Autodesk Inventor part; units mm, degrees
(part 4 of 4)
sketch "Эскиз11" plane through (0, 0, 5) normal (0, 0, 1) x (1, 0, 0)
  arc A0 (11.5664, -69.6508) -> (10.9056, -66.9499) centre (8.6538, -68.9321) ccw projected
  line L0 (10.9056, -66.9499) -> (4.435, -59.5991) projected
  arc A1 (-1.9751, -43.3567) -> (4.435, -59.5991) centre (23.7634, -42.5851) ccw projected
  arc A2 (-1.9751, -43.3567) -> (-21.6517, -33.9507) centre (-14.2373, -43.7243) ccw projected
  line L1 (-21.6517, -33.9507) -> (-22.2304, -34.418) projected
  line L2 (-22.2304, -34.418) -> (-22.7798, -34.9196) projected
  line L3 (-22.7798, -34.9196) -> (-23.0908, -35.1013) projected
  line L4 (-23.0908, -35.1013) -> (-23.2505, -35.1358) projected
  line L5 (-23.2505, -35.1358) -> (-23.3841, -35.1446) projected
  line L6 (-23.3841, -35.1446) -> (-23.5038, -35.1394) projected
  line L7 (-23.5038, -35.1394) -> (-23.6142, -35.1248) projected
  line L8 (-23.6142, -35.1248) -> (-23.8163, -35.0762) projected
  line L9 (-23.8163, -35.0762) -> (-24.0007, -35.009) projected
  line L10 (-24.0007, -35.009) -> (-24.1723, -34.9279) projected
  line L11 (-24.1723, -34.9279) -> (-24.3338, -34.8356) projected
  line L12 (-24.3338, -34.8356) -> (-24.6327, -34.6238) projected
  line L13 (-24.6327, -34.6238) -> (-24.9117, -34.3895) projected
  line L14 (-24.9117, -34.3895) -> (-25.2322, -34.2029) projected
  line L15 (-25.2322, -34.2029) -> (-25.5801, -34.0488) projected
  line L16 (-25.5801, -34.0488) -> (-25.9481, -33.9199) projected
  line L17 (-25.9481, -33.9199) -> (-26.3331, -33.8136) projected
  line L18 (-26.3331, -33.8136) -> (-26.733, -33.7285) projected
  line L19 (-26.733, -33.7285) -> (-27.1462, -33.664) projected
  line L20 (-27.1462, -33.664) -> (-27.5715, -33.6196) projected
  line L21 (-27.5715, -33.6196) -> (-28.0079, -33.5952) projected
  line L22 (-28.0079, -33.5952) -> (-28.4544, -33.5907) projected
  line L23 (-28.4544, -33.5907) -> (-28.7953, -33.6003) projected
  line L24 (-28.7953, -33.6003) -> (-29.9133, -35.4362) projected
  line L25 (-29.9133, -35.4362) -> (-29.7654, -35.7435) projected
  line L26 (-29.7654, -35.7435) -> (-29.5565, -36.138) projected
  line L27 (-29.5565, -36.138) -> (-29.3345, -36.5146) projected
  line L28 (-29.3345, -36.5146) -> (-29.0999, -36.8721) projected
  line L29 (-29.0999, -36.8721) -> (-28.8529, -37.2096) projected
  line L30 (-28.8529, -37.2096) -> (-28.5939, -37.5259) projected
  line L31 (-28.5939, -37.5259) -> (-28.3227, -37.8191) projected
  line L32 (-28.3227, -37.8191) -> (-28.0393, -38.087) projected
  line L33 (-28.0393, -38.087) -> (-27.7427, -38.3253) projected
  line L34 (-27.7427, -38.3253) -> (-27.4298, -38.5244) projected
  line L35 (-27.4298, -38.5244) -> (-27.0936, -38.6648) projected
  line L36 (-27.0936, -38.6648) -> (-26.7683, -38.8331) projected
  line L37 (-26.7683, -38.8331) -> (-26.6121, -38.9343) projected
  line L38 (-26.6121, -38.9343) -> (-26.4613, -39.0495) projected
  line L39 (-26.4613, -39.0495) -> (-26.317, -39.1826) projected
  line L40 (-26.317, -39.1826) -> (-26.1811, -39.3398) projected
  line L41 (-26.1811, -39.3398) -> (-26.1175, -39.4312) projected
  line L42 (-26.1175, -39.4312) -> (-26.0579, -39.5351) projected
  line L43 (-26.0579, -39.5351) -> (-26.0044, -39.6579) projected
  line L44 (-26.0044, -39.6579) -> (-25.9617, -39.8156) projected
  line L45 (-25.9617, -39.8156) -> (-25.9805, -40.1753) projected
  line L46 (-25.9805, -40.1753) -> (-26.174, -40.8936) projected
  line L47 (-26.174, -40.8936) -> (-26.3236, -41.6223) projected
  line L48 (-26.3236, -41.6223) -> (-26.4684, -41.9521) projected
  line L49 (-26.4684, -41.9521) -> (-26.5773, -42.0739) projected
  line L50 (-26.5773, -42.0739) -> (-26.6803, -42.1595) projected
  line L51 (-26.6803, -42.1595) -> (-26.7801, -42.2256) projected
  line L52 (-26.7801, -42.2256) -> (-26.878, -42.2788) projected
  line L53 (-26.878, -42.2788) -> (-27.0701, -42.3582) projected
  line L54 (-27.0701, -42.3582) -> (-27.2588, -42.4123) projected
  line L55 (-27.2588, -42.4123) -> (-27.4453, -42.4475) projected
  line L56 (-27.4453, -42.4475) -> (-27.6302, -42.4678) projected
  line L57 (-27.6302, -42.4678) -> (-27.9965, -42.4721) projected
  line L58 (-27.9965, -42.4721) -> (-28.3599, -42.4466) projected
  line L59 (-28.3599, -42.4466) -> (-28.7289, -42.484) projected
  line L60 (-28.7289, -42.484) -> (-29.101, -42.5638) projected
  line L61 (-29.101, -42.5638) -> (-29.4745, -42.6758) projected
  line L62 (-29.4745, -42.6758) -> (-29.8484, -42.8161) projected
  line L63 (-29.8484, -42.8161) -> (-30.2219, -42.9823) projected
  line L64 (-30.2219, -42.9823) -> (-30.5941, -43.173) projected
  line L65 (-30.5941, -43.173) -> (-30.9643, -43.3871) projected
  line L66 (-30.9643, -43.3871) -> (-31.3317, -43.6239) projected
  line L67 (-31.3317, -43.6239) -> (-31.6956, -43.8826) projected
  line L68 (-31.6956, -43.8826) -> (-31.9658, -44.0908) projected
  line L69 (-31.9658, -44.0908) -> (-31.7912, -46.2332) projected
  line L70 (-31.7912, -46.2332) -> (-31.4909, -46.3949) projected
  line L71 (-31.4909, -46.3949) -> (-31.0899, -46.5913) projected
  line L72 (-31.0899, -46.5913) -> (-30.689, -46.7654) projected
  line L73 (-30.689, -46.7654) -> (-30.289, -46.9168) projected
  line L74 (-30.289, -46.9168) -> (-29.8909, -47.0447) projected
  line L75 (-29.8909, -47.0447) -> (-29.4954, -47.1483) projected
  line L76 (-29.4954, -47.1483) -> (-29.1037, -47.2261) projected
  line L77 (-29.1037, -47.2261) -> (-28.7169, -47.2762) projected
  line L78 (-28.7169, -47.2762) -> (-28.3369, -47.2947) projected
  line L79 (-28.3369, -47.2947) -> (-27.9667, -47.2719) projected
  line L80 (-27.9667, -47.2719) -> (-27.6122, -47.1878) projected
  line L81 (-27.6122, -47.1878) -> (-27.2501, -47.1328) projected
  line L82 (-27.2501, -47.1328) -> (-27.0643, -47.1228) projected
  line L83 (-27.0643, -47.1228) -> (-26.8745, -47.1274) projected
  line L84 (-26.8745, -47.1274) -> (-26.6796, -47.1502) projected
  line L85 (-26.6796, -47.1502) -> (-26.4772, -47.1975) projected
  line L86 (-26.4772, -47.1975) -> (-26.372, -47.2341) projected
  line L87 (-26.372, -47.2341) -> (-26.2627, -47.2832) projected
  line L88 (-26.2627, -47.2832) -> (-26.1473, -47.351) projected
  line L89 (-26.1473, -47.351) -> (-26.0201, -47.4535) projected
  line L90 (-26.0201, -47.4535) -> (-25.8238, -47.7556) projected
  line L91 (-25.8238, -47.7556) -> (-25.5582, -48.4504) projected
  line L92 (-25.5582, -48.4504) -> (-25.2509, -49.1279) projected
  line L93 (-25.2509, -49.1279) -> (-25.1742, -49.4799) projected
  line L94 (-25.1742, -49.4799) -> (-25.1907, -49.6424) projected
  line L95 (-25.1907, -49.6424) -> (-25.2237, -49.7722) projected
  line L96 (-25.2237, -49.7722) -> (-25.2656, -49.8844) projected
  line L97 (-25.2656, -49.8844) -> (-25.3136, -49.9849) projected
  line L98 (-25.3136, -49.9849) -> (-25.4222, -50.1621) projected
  line L99 (-25.4222, -50.1621) -> (-25.5431, -50.3167) projected
  line L100 (-25.5431, -50.3167) -> (-25.6733, -50.4549) projected
  line L101 (-25.6733, -50.4549) -> (-25.811, -50.58) projected
  line L102 (-25.811, -50.58) -> (-26.1047, -50.7987) projected
  line L103 (-26.1047, -50.7987) -> (-26.4138, -50.9917) projected
  line L104 (-26.4138, -50.9917) -> (-26.6903, -51.2389) projected
  line L105 (-26.6903, -51.2389) -> (-26.9445, -51.5221) projected
  line L106 (-26.9445, -51.5221) -> (-27.1808, -51.8323) projected
  line L107 (-27.1808, -51.8323) -> (-27.4008, -52.1655) projected
  line L108 (-27.4008, -52.1655) -> (-27.6053, -52.5195) projected
  line L109 (-27.6053, -52.5195) -> (-27.7943, -52.8926) projected
  line L110 (-27.7943, -52.8926) -> (-27.968, -53.2834) projected
  line L111 (-27.968, -53.2834) -> (-28.126, -53.6909) projected
  line L112 (-28.126, -53.6909) -> (-28.2683, -54.1141) projected
  line L113 (-28.2683, -54.1141) -> (-28.3645, -54.4413) projected
  line L114 (-28.3645, -54.4413) -> (-26.964, -56.072) projected
  line L115 (-26.964, -56.072) -> (-26.626, -56.0262) projected
  line L116 (-26.626, -56.0262) -> (-26.1862, -55.9495) projected
  line L117 (-26.1862, -55.9495) -> (-25.7595, -55.8547) projected
  line L118 (-25.7595, -55.8547) -> (-25.347, -55.7421) projected
  line L119 (-25.347, -55.7421) -> (-24.9496, -55.6115) projected
  line L120 (-24.9496, -55.6115) -> (-24.5688, -55.4628) projected
  line L121 (-24.5688, -55.4628) -> (-24.2061, -55.2956) projected
  line L122 (-24.2061, -55.2956) -> (-23.8638, -55.1088) projected
  line L123 (-23.8638, -55.1088) -> (-23.5455, -54.9003) projected
  line L124 (-23.5455, -54.9003) -> (-23.2594, -54.6643) projected
  line L125 (-23.2594, -54.6643) -> (-23.022, -54.3879) projected
  line L126 (-23.022, -54.3879) -> (-22.7614, -54.1305) projected
  line L127 (-22.7614, -54.1305) -> (-22.617, -54.0133) projected
  line L128 (-22.617, -54.0133) -> (-22.4608, -53.9055) projected
  line L129 (-22.4608, -53.9055) -> (-22.2896, -53.8093) projected
  line L130 (-22.2896, -53.8093) -> (-22.0981, -53.7286) projected
  line L131 (-22.0981, -53.7286) -> (-21.9915, -53.6964) projected
  line L132 (-21.9915, -53.6964) -> (-21.8742, -53.6719) projected
  line L133 (-21.8742, -53.6719) -> (-21.741, -53.6589) projected
  line L134 (-21.741, -53.6589) -> (-21.5778, -53.6671) projected
  line L135 (-21.5778, -53.6671) -> (-21.2415, -53.7961) projected
  line L136 (-21.2415, -53.7961) -> (-20.6181, -54.2021) projected
  line L137 (-20.6181, -54.2021) -> (-19.9714, -54.5696) projected
  line L138 (-19.9714, -54.5696) -> (-19.7024, -54.8092) projected
  line L139 (-19.7024, -54.8092) -> (-19.6203, -54.9504) projected
  line L140 (-19.6203, -54.9504) -> (-19.5706, -55.0748) projected
  line L141 (-19.5706, -55.0748) -> (-19.5386, -55.1902) projected
  line L142 (-19.5386, -55.1902) -> (-19.5183, -55.2997) projected
  line L143 (-19.5183, -55.2997) -> (-19.5021, -55.5069) projected
  line L144 (-19.5021, -55.5069) -> (-19.509, -55.7031) projected
  line L145 (-19.509, -55.7031) -> (-19.5331, -55.8914) projected
  line L146 (-19.5331, -55.8914) -> (-19.571, -56.0735) projected
  line L147 (-19.571, -56.0735) -> (-19.68, -56.4231) projected
  line L148 (-19.68, -56.4231) -> (-19.8167, -56.7609) projected
  line L149 (-19.8167, -56.7609) -> (-19.8951, -57.1234) projected
  line L150 (-19.8951, -57.1234) -> (-19.9342, -57.5019) projected
  line L151 (-19.9342, -57.5019) -> (-19.9431, -57.8918) projected
  line L152 (-19.9431, -57.8918) -> (-19.9252, -58.2907) projected
  line L153 (-19.9252, -58.2907) -> (-19.8825, -58.6973) projected
  line L154 (-19.8825, -58.6973) -> (-19.8162, -59.1102) projected
  line L155 (-19.8162, -59.1102) -> (-19.7269, -59.5285) projected
  line L156 (-19.7269, -59.5285) -> (-19.6153, -59.9511) projected
  line L157 (-19.6153, -59.9511) -> (-19.4817, -60.3771) projected
  line L158 (-19.4817, -60.3771) -> (-19.3672, -60.6983) projected
  line L159 (-19.3672, -60.6983) -> (-17.2757, -61.1943) projected
  line L160 (-17.2757, -61.1943) -> (-17.0291, -60.9587) projected
  line L161 (-17.0291, -60.9587) -> (-16.7184, -60.6381) projected
  line L162 (-16.7184, -60.6381) -> (-16.4289, -60.3106) projected
  line L163 (-16.4289, -60.3106) -> (-16.1614, -59.977) projected
  line L164 (-16.1614, -59.977) -> (-15.9167, -59.6378) projected
  line L165 (-15.9167, -59.6378) -> (-15.696, -59.2937) projected
  line L166 (-15.696, -59.2937) -> (-15.5009, -58.9452) projected
  line L167 (-15.5009, -58.9452) -> (-15.3337, -58.5929) projected
  line L168 (-15.3337, -58.5929) -> (-15.1987, -58.2372) projected
  line L169 (-15.1987, -58.2372) -> (-15.106, -57.878) projected
  line L170 (-15.106, -57.878) -> (-15.0764, -57.5149) projected
  line L171 (-15.0764, -57.5149) -> (-15.0169, -57.1535) projected
  line L172 (-15.0169, -57.1535) -> (-14.9689, -56.9737) projected
  line L173 (-14.9689, -56.9737) -> (-14.9059, -56.7947) projected
  line L174 (-14.9059, -56.7947) -> (-14.824, -56.6163) projected
  line L175 (-14.824, -56.6163) -> (-14.7164, -56.4385) projected
  line L176 (-14.7164, -56.4385) -> (-14.6491, -56.3497) projected
  line L177 (-14.6491, -56.3497) -> (-14.5687, -56.261) projected
  line L178 (-14.5687, -56.261) -> (-14.4685, -56.1721) projected
  line L179 (-14.4685, -56.1721) -> (-14.3317, -56.0828) projected
  line L180 (-14.3317, -56.0828) -> (-13.9838, -55.9895) projected
  line L181 (-13.9838, -55.9895) -> (-13.2409, -55.9516) projected
  line L182 (-13.2409, -55.9516) -> (-12.5016, -55.8687) projected
  arc A3 (4.4993, -64.4993) -> (-12.5016, -55.8687) centre (-14.8291, -81.5133) ccw projected
  line L183 (4.4993, -64.4993) -> (7.5502, -67.9652) projected
  arc A4 (8.211, -70.6661) -> (7.5502, -67.9652) centre (5.2984, -69.9474) ccw projected
  line L184 (8.211, -70.6661) -> (3.0154, -91.7239) projected
  line L185 (3.0154, -91.7239) -> (6.1993, -91.4035) projected
  line L186 (6.1993, -91.4035) -> (11.5664, -69.6508) projected
  circle A5 centre (-14.2373, -43.7243) radius 2.5 projected
  circle A6 centre (-8.2184, -38.4544) radius 1.6 projected
  circle A7 centre (-19.5073, -37.7054) radius 1.6 projected
  circle A8 centre (-20.2562, -48.9943) radius 1.6 projected
  circle A9 centre (-8.9673, -49.7433) radius 1.6 projected
  circle A10 centre (-39.9568, -59.168) radius 2.5 projected
  line L187 (-14.2373, -43.7243) -> (-39.9568, -59.168)
  line L188 (-27.0971, -51.4462) -> (-13.5779, -73.9607)
  arc A11 (-31.273, -92.2767) -> (-29.1996, -94.1293) centre (-28.4651, -91.2206) ccw
  line L189 (-31.273, -92.2767) -> (-34.7203, -83.1105)
  arc A12 (-34.7203, -83.1105) -> (-46.0444, -69.8188) centre (-58.8222, -92.1748) ccw
  arc A13 (-30.0531, -66.4077) -> (-30.4253, -85.4702) centre (-6.3234, -76.4059) ccw
  line L190 (-30.4253, -85.4702) -> (-28.7999, -89.7922)
  arc A14 (-28.7999, -89.7922) -> (-26.7265, -91.6448) centre (-25.9919, -88.7361) ccw
  line L191 (-26.7265, -91.6448) -> (-5.6974, -96.9556)
  line L192 (-5.6974, -96.9556) -> (-7.4766, -99.6154)
  line L193 (-7.4766, -99.6154) -> (-29.1996, -94.1293)
  circle A15 centre (-47.4326, -62.0164) radius 1.6 projected
  circle A16 centre (-37.1084, -66.6437) radius 1.6 projected
  circle A17 centre (-32.4811, -56.3196) radius 1.6 projected
  circle A18 centre (-39.9568, -59.168) radius 2.5 projected
  circle A19 centre (-42.8052, -51.6922) radius 1.6 projected
  arc A20 (-41.4259, -46.9885) -> (-28.2942, -62.9735) centre (-39.9568, -59.168) ccw projected
  line L194 (-28.085, -62.2597) -> (-28.2942, -62.9735) projected
  line L195 (-27.9195, -61.5344) -> (-28.085, -62.2597) projected
  line L196 (-27.7675, -61.2078) -> (-27.9195, -61.5344) projected
  line L197 (-27.6559, -61.0885) -> (-27.7675, -61.2078) projected
  line L198 (-27.5511, -61.0052) -> (-27.6559, -61.0885) projected
  line L199 (-27.4498, -60.9413) -> (-27.5511, -61.0052) projected
  line L200 (-27.3508, -60.8903) -> (-27.4498, -60.9413) projected
  line L201 (-27.1571, -60.815) -> (-27.3508, -60.8903) projected
  line L202 (-26.9672, -60.7651) -> (-27.1571, -60.815) projected
  line L203 (-26.78, -60.734) -> (-26.9672, -60.7651) projected
  line L204 (-26.5947, -60.7178) -> (-26.78, -60.734) projected
  line L205 (-26.2284, -60.7215) -> (-26.5947, -60.7178) projected
  line L206 (-25.8656, -60.755) -> (-26.2284, -60.7215) projected
  line L207 (-25.4958, -60.7256) -> (-25.8656, -60.755) projected
  line L208 (-25.1221, -60.6541) -> (-25.4958, -60.7256) projected
  line L209 (-24.7463, -60.5502) -> (-25.1221, -60.6541) projected
  line L210 (-24.3693, -60.4182) -> (-24.7463, -60.5502) projected
  line L211 (-23.9923, -60.2602) -> (-24.3693, -60.4182) projected
  line L212 (-23.616, -60.0777) -> (-23.9923, -60.2602) projected
  line L213 (-23.2412, -59.8717) -> (-23.616, -60.0777) projected
  line L214 (-22.8687, -59.6431) -> (-23.2412, -59.8717) projected
  line L215 (-22.4992, -59.3924) -> (-22.8687, -59.6431) projected
  line L216 (-22.2246, -59.1902) -> (-22.4992, -59.3924) projected
  line L217 (-22.3522, -57.0445) -> (-22.2246, -59.1902) projected
  line L218 (-22.6489, -56.8763) -> (-22.3522, -57.0445) projected
  line L219 (-23.0454, -56.6711) -> (-22.6489, -56.8763) projected
  line L220 (-23.4424, -56.4882) -> (-23.0454, -56.6711) projected
  line L221 (-23.839, -56.3281) -> (-23.4424, -56.4882) projected
  line L222 (-24.2343, -56.1915) -> (-23.839, -56.3281) projected
  line L223 (-24.6274, -56.0793) -> (-24.2343, -56.1915) projected
  line L224 (-25.0173, -55.9929) -> (-24.6274, -56.0793) projected
  line L225 (-25.4028, -55.9343) -> (-25.0173, -55.9929) projected
  line L226 (-25.7823, -55.9075) -> (-25.4028, -55.9343) projected
  line L227 (-26.153, -55.9222) -> (-25.7823, -55.9075) projected
  line L228 (-26.5093, -55.9985) -> (-26.153, -55.9222) projected
  line L229 (-26.8725, -56.0456) -> (-26.5093, -55.9985) projected
  line L230 (-27.0584, -56.0515) -> (-26.8725, -56.0456) projected
  line L231 (-27.248, -56.0427) -> (-27.0584, -56.0515) projected
  line L232 (-27.4425, -56.0157) -> (-27.248, -56.0427) projected
  line L233 (-27.6437, -55.9639) -> (-27.4425, -56.0157) projected
  line L234 (-27.7481, -55.925) -> (-27.6437, -55.9639) projected
  line L235 (-27.8563, -55.8736) -> (-27.7481, -55.925) projected
  line L236 (-27.9702, -55.8032) -> (-27.8563, -55.8736) projected
  line L237 (-28.0951, -55.698) -> (-27.9702, -55.8032) projected
  line L238 (-28.2847, -55.3917) -> (-28.0951, -55.698) projected
  line L239 (-28.5351, -54.6912) -> (-28.2847, -55.3917) projected
  line L240 (-28.8274, -54.0071) -> (-28.5351, -54.6912) projected
  line L241 (-28.8965, -53.6536) -> (-28.8274, -54.0071) projected
  line L242 (-28.8763, -53.4914) -> (-28.8965, -53.6536) projected
  line L243 (-28.8405, -53.3624) -> (-28.8763, -53.4914) projected
  line L244 (-28.7962, -53.2512) -> (-28.8405, -53.3624) projected
  line L245 (-28.746, -53.1517) -> (-28.7962, -53.2512) projected
  line L246 (-28.6335, -52.977) -> (-28.746, -53.1517) projected
  line L247 (-28.5092, -52.825) -> (-28.6335, -52.977) projected
  line L248 (-28.3761, -52.6897) -> (-28.5092, -52.825) projected
  line L249 (-28.2357, -52.5677) -> (-28.3761, -52.6897) projected
  line L250 (-27.9372, -52.3554) -> (-28.2357, -52.5677) projected
  line L251 (-27.624, -52.1693) -> (-27.9372, -52.3554) projected
  line L252 (-27.3421, -51.9282) -> (-27.624, -52.1693) projected
  line L253 (-27.0818, -51.6507) -> (-27.3421, -51.9282) projected
  line L254 (-26.8388, -51.3457) -> (-27.0818, -51.6507) projected
  line L255 (-26.6114, -51.0173) -> (-26.8388, -51.3457) projected
  line L256 (-26.3993, -50.6679) -> (-26.6114, -51.0173) projected
  line L257 (-26.2021, -50.2991) -> (-26.3993, -50.6679) projected
  line L258 (-26.02, -49.9121) -> (-26.2021, -50.2991) projected
  line L259 (-25.853, -49.5082) -> (-26.02, -49.9121) projected
  line L260 (-25.7014, -49.0882) -> (-25.853, -49.5082) projected
  line L261 (-25.5981, -48.7632) -> (-25.7014, -49.0882) projected
  line L262 (-25.5981, -48.7632) -> (-26.9625, -47.1023) projected
  line L263 (-27.3014, -47.1406) -> (-26.9625, -47.1023) projected
  line L264 (-27.7429, -47.2077) -> (-27.3014, -47.1406) projected
  line L265 (-28.1715, -47.2931) -> (-27.7429, -47.2077) projected
  line L266 (-28.5864, -47.3967) -> (-28.1715, -47.2931) projected
  line L267 (-28.9865, -47.5185) -> (-28.5864, -47.3967) projected
  line L268 (-29.3705, -47.6588) -> (-28.9865, -47.5185) projected
  line L269 (-29.7368, -47.818) -> (-29.3705, -47.6588) projected
  line L270 (-30.0831, -47.9973) -> (-29.7368, -47.818) projected
  line L271 (-30.4059, -48.1987) -> (-30.0831, -47.9973) projected
  line L272 (-30.6971, -48.4284) -> (-30.4059, -48.1987) projected
  line L273 (-30.9405, -48.6995) -> (-30.6971, -48.4284) projected
  line L274 (-31.2067, -48.9511) -> (-30.9405, -48.6995) projected
  line L275 (-31.3536, -49.0652) -> (-31.2067, -48.9511) projected
  line L276 (-31.5122, -49.1695) -> (-31.3536, -49.0652) projected
  line L277 (-31.6854, -49.262) -> (-31.5122, -49.1695) projected
  line L278 (-31.8786, -49.3384) -> (-31.6854, -49.262) projected
  line L279 (-31.986, -49.3683) -> (-31.8786, -49.3384) projected
  line L280 (-32.1037, -49.3902) -> (-31.986, -49.3683) projected
  line L281 (-32.2372, -49.4003) -> (-32.1037, -49.3902) projected
  line L282 (-32.4002, -49.3886) -> (-32.2372, -49.4003) projected
  line L283 (-32.7336, -49.2522) -> (-32.4002, -49.3886) projected
  line L284 (-33.3479, -48.8326) -> (-32.7336, -49.2522) projected
  line L285 (-33.9864, -48.4511) -> (-33.3479, -48.8326) projected
  line L286 (-34.2501, -48.2056) -> (-33.9864, -48.4511) projected
  line L287 (-34.3291, -48.0626) -> (-34.2501, -48.2056) projected
  line L288 (-34.376, -47.9372) -> (-34.3291, -48.0626) projected
  line L289 (-34.4055, -47.8211) -> (-34.376, -47.9372) projected
  line L290 (-34.4234, -47.7112) -> (-34.4055, -47.8211) projected
  line L291 (-34.4351, -47.5037) -> (-34.4234, -47.7112) projected
  line L292 (-34.4238, -47.3077) -> (-34.4351, -47.5037) projected
  line L293 (-34.3956, -47.12) -> (-34.4238, -47.3077) projected
  line L294 (-34.3538, -46.9387) -> (-34.3956, -47.12) projected
  line L295 (-34.237, -46.5916) -> (-34.3538, -46.9387) projected
  line L296 (-34.0931, -46.2568) -> (-34.237, -46.5916) projected
  line L297 (-34.0067, -45.8961) -> (-34.0931, -46.2568) projected
  line L298 (-33.9593, -45.5186) -> (-34.0067, -45.8961) projected
  line L299 (-33.9419, -45.129) -> (-33.9593, -45.5186) projected
  line L300 (-33.951, -44.7298) -> (-33.9419, -45.129) projected
  line L301 (-33.9848, -44.3224) -> (-33.951, -44.7298) projected
  line L302 (-34.0421, -43.9081) -> (-33.9848, -44.3224) projected
  line L303 (-34.1221, -43.488) -> (-34.0421, -43.9081) projected
  line L304 (-34.2244, -43.063) -> (-34.1221, -43.488) projected
  line L305 (-34.3487, -42.6342) -> (-34.2244, -43.063) projected
  line L306 (-34.4561, -42.3105) -> (-34.3487, -42.6342) projected
  line L307 (-36.5363, -41.7688) -> (-34.4561, -42.3105) projected
  line L308 (-36.7879, -41.999) -> (-36.5363, -41.7688) projected
  line L309 (-37.1056, -42.3127) -> (-36.7879, -41.999) projected
  line L310 (-37.4022, -42.6338) -> (-37.1056, -42.3127) projected
  line L311 (-37.677, -42.9614) -> (-37.4022, -42.6338) projected
  line L312 (-37.9291, -43.2952) -> (-37.677, -42.9614) projected
  line L313 (-38.1573, -43.6344) -> (-37.9291, -43.2952) projected
  line L314 (-38.36, -43.9785) -> (-38.1573, -43.6344) projected
  line L315 (-38.5348, -44.327) -> (-38.36, -43.9785) projected
  line L316 (-38.6775, -44.6797) -> (-38.5348, -44.327) projected
  line L317 (-38.7781, -45.0367) -> (-38.6775, -44.6797) projected
  line L318 (-38.8157, -45.3992) -> (-38.7781, -45.0367) projected
  line L319 (-38.8831, -45.7592) -> (-38.8157, -45.3992) projected
  line L320 (-38.935, -45.9378) -> (-38.8831, -45.7592) projected
  line L321 (-39.0019, -46.1155) -> (-38.935, -45.9378) projected
  line L322 (-39.0877, -46.292) -> (-39.0019, -46.1155) projected
  line L323 (-39.1991, -46.4674) -> (-39.0877, -46.292) projected
  line L324 (-39.2684, -46.5547) -> (-39.1991, -46.4674) projected
  line L325 (-39.3507, -46.6417) -> (-39.2684, -46.5547) projected
  line L326 (-39.4528, -46.7283) -> (-39.3507, -46.6417) projected
  line L327 (-39.5916, -46.8146) -> (-39.4528, -46.7283) projected
  line L328 (-39.9414, -46.9002) -> (-39.5916, -46.8146) projected
  line L329 (-40.685, -46.9219) -> (-39.9414, -46.9002) projected
  line L330 (-41.4259, -46.9885) -> (-40.685, -46.9219) projected
  point P0 (0, 0)
  point P1 (-30.0531, -66.4077)
  point P2 (-46.0397, -69.8215)
  constraints: 14 end point, 14 symmetric about line, 8 point on circle, 4 centre point, 1 midpoint, 1 perpendicular, 4 other
extrude "Выдавливание11" add sketch "Эскиз11" against normal up to surface (5 mm away) contours A13 L190 A14 L191 L192 L193 A11 L189 A12 A20
